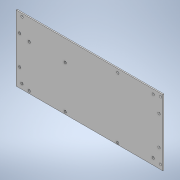
# Autodesk Inventor part: 20220624_知能ロボット2階部分
Saved by Autodesk Inventor 2020 (Build 240168000, 168)
## iProperties
Created: 2022-06-24
Part Number: 20220624_知能ロボット2階部分
Material: 一般
Document SubType Name: Modeling
Designer: Naggy
Density: 1 g/cm^3
Appearance: 既定
Author: Naggy
Autodesk Inventor part; units mm, degrees
ref_plane "YZ Plane" through (0, 0, 0) normal (1, 0, 0) x (0, 1, 0)
ref_plane "XZ Plane" through (0, 0, 0) normal (0, 1, 0) x (-1, 0, 0)
ref_plane "XY Plane" through (0, 0, 0) normal (0, 0, 1) x (1, 0, 0)
sketch "スケッチ1" plane through (0, 0, 0) normal (0, 0, 1) x (1, 0, 0)
  line L0 (-100, -45) -> (100, -45)
  line L1 (100, -45) -> (100, 45)
  line L2 (100, 45) -> (-100, 45)
  line L3 (-100, 45) -> (-100, -45)
  line L4 (-100, -45) -> (100, 45) construction
  line L5 (100, -45) -> (-100, 45) construction
  point P0 (0, 0)
  dimension "d0" = 200
  dimension "d1" = 90
  constraints: 12 end point, 2 midpoint, 2 parallel, 1 horizontal, 1 perpendicular
  measures "d0" distance between parallel lines of L1 L3
  measures "d1" distance between parallel lines of L0 L2
extrude "押し出し1" add sketch "スケッチ1" along normal blind 1.5
sketch "スケッチ2" plane through (0, 0, 1.5) normal (0, 0, 1) x (1, 0, 0)
  line L0 (100, -45) -> (100, 45) projected
  line L1 (-100, -45) -> (100, -45) projected
  point P0 (0, 0)
  point P1 (97, 41)
  point P2 (97, -39)
  dimension "d4" = 3
  dimension "d5" = 3
  dimension "d6" = 6
  dimension "d7" = 86
  measures "d4" distance from line of point (97, 41) L0
  measures "d5" distance from line of point (97, -39) L0
  measures "d6" distance from line of L1 point (97, -39)
  measures "d7" distance from line of L1 point (97, 41)
hole "穴1" at (97, 41, 1.5) at (97, -39, 1.5) direction (0, 0, -1) diameter 3.2 depth 8.8 tip angle 118
sketch "スケッチ3" plane through (0, 0, 1.5) normal (0, 0, 1) x (1, 0, 0)
  line L0 (-100, 45) -> (-100, -45) projected
  line L1 (-100, -45) -> (100, -45) projected
  point P0 (0, 0)
  point P1 (-92, 41)
  point P2 (-92, -38)
  dimension "d15" = 8
  dimension "d16" = 8
  dimension "d17" = 7
  dimension "d18" = 86
  measures "d15" distance from line of point (-92, 41) L0
  measures "d16" distance from line of point (-92, -38) L0
  measures "d17" distance from line of L1 point (-92, -38)
  measures "d18" distance from line of point (-92, 41) L1
hole "穴2" at (-92, 41, 1.5) at (-92, -38, 1.5) direction (0, 0, -1) diameter 3.2 depth 8.8 tip angle 118
sketch "スケッチ4" plane through (0, 0, 1.5) normal (0, 0, 1) x (1, 0, 0)
  circle A0 centre (97, -39) radius 1.6 projected
  line L0 (-100, -45) -> (100, -45) projected
  line L1 (100, -45) -> (100, 45) projected
  circle A1 centre (97, 41) radius 1.6 projected
  point P0 (0, 0)
  point P1 (87, 38.82)
  point P2 (87, -36.11)
  dimension "d26" = 10
  dimension "d27" = 8.89
  dimension "d29" = 74.93
  dimension "d41" = 10
  measures "d26" horizontal distance of point (87, -36.11) A0.centre
  measures "d27" distance from line of point (87, -36.11) L0
  measures "d29" distance of point (87, 38.82) point (87, -36.11)
  measures "d41" horizontal distance of point (87, 38.82) A1.centre
hole "穴3" at (87, 38.82, 1.5) at (87, -36.11, 1.5) direction (0, 0, -1) diameter 3.2 depth 8.8 tip angle 118
sketch "スケッチ10" plane through (0, 0, 1.5) normal (0, 0, 1) x (1, 0, 0)
  circle A0 centre (87, -36.11) radius 1.6 projected
  line L0 (-100, -45) -> (100, -45) projected
  circle A1 centre (87, 38.82) radius 1.6 projected
  point P0 (0, 0)
  point P1 (38.74, 40.09)
  point P2 (38.74, -42.46)
  dimension "d43" = 2.54
  dimension "d44" = 48.26
  dimension "d46" = 82.55
  measures "d43" distance from line of point (38.74, -42.46) L0
  measures "d44" horizontal distance of point (38.74, -42.46) A0.centre
  measures "d46" distance of point (38.74, 40.09) point (38.74, -42.46)
hole "穴4" at (38.74, 40.09, 1.5) at (38.74, -42.46, 1.5) direction (0, 0, -1) diameter 3.2 depth 8.8 tip angle 118
sketch "スケッチ11" plane through (0, 0, 1.5) normal (0, 0, 1) x (1, 0, 0)
  line L0 (-100, -45) -> (100, -45) projected
  circle A0 centre (-92, -38) radius 1.6 projected
  point P0 (0, 0)
  point P1 (-82, 16.5)
  point P2 (-33, 16.5)
  point P3 (-33, -41.5)
  point P4 (-82, -41.5)
  dimension "d54" = 3.5
  dimension "d55" = 3.5
  dimension "d56" = 10
  dimension "d57" = 49
  dimension "d58" = 10
  dimension "d59" = 58
  dimension "d60" = 58
  dimension "d61" = 49
  measures "d54" distance from line of point (-82, -41.5) L0
  measures "d55" distance from line of point (-33, -41.5) L0
  measures "d56" horizontal distance of point (-82, -41.5) A0.centre
  measures "d57" distance of point (-33, -41.5) point (-82, -41.5)
  measures "d58" horizontal distance of A0.centre point (-82, 16.5)
  measures "d59" distance of point (-82, 16.5) point (-82, -41.5)
  measures "d60" distance of point (-33, 16.5) point (-33, -41.5)
  measures "d61" distance of point (-33, 16.5) point (-82, 16.5)
hole "穴5" at (-82, 16.5, 1.5) at (-33, 16.5, 1.5) at (-33, -41.5, 1.5) at (-82, -41.5, 1.5) direction (0, 0, -1) diameter 3.2 depth 8.8 tip angle 118
sketch "スケッチ12" plane through (0, 0, 1.5) normal (0, 0, 1) x (1, 0, 0)
  line L0 (-100, 45) -> (-100, -45) projected
  line L1 (100, 45) -> (-100, 45) projected
  line L2 (-100, -45) -> (100, -45) projected
  line L3 (100, -45) -> (100, 45) projected
  point P0 (0, 0)
  point P1 (-95, 20)
  point P2 (-95, -20)
  point P3 (95, 20)
  point P4 (95, -20)
  dimension "d69" = 5
  dimension "d70" = 25
  dimension "d71" = 5
  dimension "d72" = 25
  dimension "d73" = 5
  dimension "d74" = 5
  measures "d69" distance from line of point (-95, 20) L0
  measures "d70" distance from line of point (-95, 20) L1
  measures "d71" distance from line of point (-95, -20) L0
  measures "d72" distance from line of point (-95, -20) L2
  measures "d73" distance from line of point (95, -20) L3
  measures "d74" distance from line of point (95, 20) L3
hole "穴6" at (-95, 20, 1.5) at (-95, -20, 1.5) at (95, 20, 1.5) at (95, -20, 1.5) direction (0, 0, -1) diameter 3.2 depth 8.8 tip angle 118
